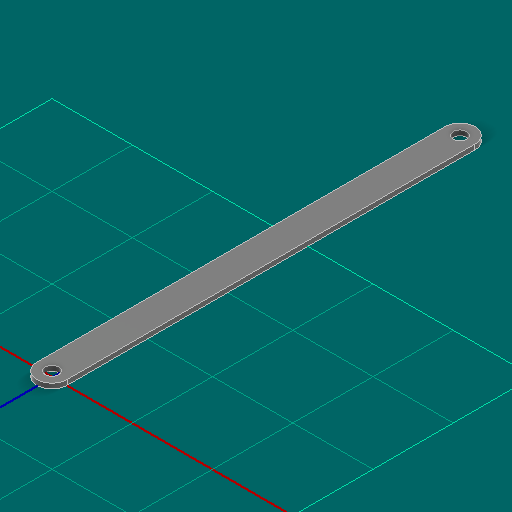
# Autodesk Inventor part: brace-gussest
Saved by Autodesk Inventor 2025 (Build 290162000, 162)
## iProperties
Created: 2024-08-11
Part Number: brace-gussest
Material: Acetal Resin, Black
Document SubType Name: Sheet Metal
Designer: averey
Density: 1.425 g/cm^3
Sheet Metal Rule: Default
Appearance: Smooth - Black
Author: averey
Autodesk Inventor part; units mm, degrees
ref_plane "YZ Plane" through (0, 0, 0) normal (1, 0, 0) x (0, 1, 0)
ref_plane "XZ Plane" through (0, 0, 0) normal (0, 1, 0) x (-1, 0, 0)
ref_plane "XY Plane" through (0, 0, 0) normal (0, 0, 1) x (1, 0, 0)
sketch "Sketch1" plane through (0, 0, 0) normal (0, 1, 0) x (-1, 0, 0)
  circle A0 centre (0, 0) radius 2.0955
  circle A1 centre (0, -129.1082) radius 2.0955
  arc A2 (4.7625, 0) -> (-4.7625, 0) centre (0, 0) ccw
  arc A3 (-4.7625, -129.1082) -> (4.7625, -129.1082) centre (0, -129.1082) ccw
  line L0 (4.7625, 0) -> (4.7625, -129.1082)
  line L1 (-4.7625, -129.1082) -> (-4.7625, 0)
  dimension "d0" = 4.191
  dimension "d1" = 4.191
  dimension "d2" = 9.525
  dimension "d3" = 9.525
  constraints: 4 centre point, 4 end point, 4 point on circle, 3 coincident, 3 tangent
  measures "d0" diameter of A0
  measures "d1" diameter of A1
  measures "d2" diameter of A2
  measures "d3" diameter of A3
extrude "Extrusion1" add sketch "Sketch1" along normal blind 1.5875
equation "\"BendRadius\" = Thickness"
equation "\"BendReliefWidth\" = Thickness"
equation "\"BendReliefDepth\" = 0.5 * Thickness"
equation "\"CornerReliefSize\" = 4 * Thickness"
equation "\"MinimumRemnant\" = 2 * Thickness"
equation "\"TransitionRadius\" = BendRadius"
equation "\"JacobiRadiusSize\" = BendRadius"
equation "\"GapSize\" = Thickness"
equation "\"Thickness\" = 3.048"
body "Solid1"
